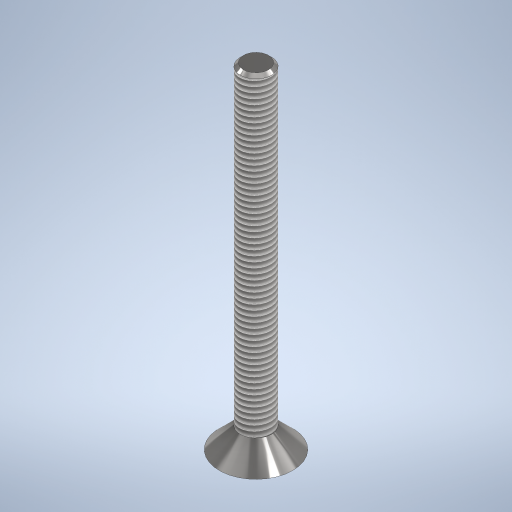
# Autodesk Inventor part: M3 30mm 십자나사
Saved by Autodesk Inventor 2023 (Build 270158000, 158)
## iProperties
Created: 2022-06-21
Part Number: M3 30mm 십자나사
Material: 일반
Document SubType Name: Modeling
Designer: user
Density: 1 g/cm^3
Appearance: 기본값
Author: user
Autodesk Inventor part; units mm, degrees
ref_plane "YZ Plane" through (0, 0, 0) normal (1, 0, 0) x (0, 1, 0)
ref_plane "XZ Plane" through (0, 0, 0) normal (0, 1, 0) x (-1, 0, 0)
ref_plane "XY Plane" through (0, 0, 0) normal (0, 0, 1) x (1, 0, 0)
sketch "스케치1" plane through (0, 0, 0) normal (0, 0, 1) x (1, 0, 0)
  line L0 (0, 0) -> (0, 30)
  line L1 (0, 30) -> (1.5, 30)
  line L2 (1.5, 30) -> (1.5, 0)
  line L3 (0, -2) -> (3.5, -2)
  line L4 (3.5, -2) -> (1.5, 0)
  line L5 (0, 0) -> (0, -2)
  dimension "d0" = 30
  dimension "d1" = 7
  dimension "d2" = 3
  dimension "d3" = 45
  constraints: 12 end point, 2 perpendicular, 2 vertical, 1 horizontal, 1 horizontal alignment
  measures "d0" distance of L0.start L0.end
  measures "d1" diameter of L3.end L0
  measures "d2" diameter of L2 L0
  measures "d3" angle of L5 L4
revolve "회전1" add sketch "스케치1" angle 360 about axis through (0, 0, 0) along (0, 1, 0)
chamfer "모따기1" distance 0.3 angle 45 1 edges at (-1.5, 30, 0)
thread "스레드1" size "M3x0.5" class "6g" standard "ANSI Metric M Profile" full length
sketch "스케치2" plane through (0, -2, 0) normal (0, -1, 0) x (1, 0, 0)
  line L0 (-0.5, 2.5) -> (0.5, 2.5)
  line L1 (0.5, 2.5) -> (0.5, -2.5)
  line L2 (0.5, -2.5) -> (-0.5, -2.5)
  line L3 (-0.5, -2.5) -> (-0.5, 2.5)
  circle A0 centre (0, 0) radius 1.2 construction
  line L4 (-0.5, 2.5) -> (0.5, -2.5) construction
  line L5 (0.5, 2.5) -> (-0.5, -2.5) construction
  line L6 (-2.5, -0.5) -> (2.5, -0.5)
  line L7 (2.5, -0.5) -> (2.5, 0.5)
  line L8 (2.5, 0.5) -> (-2.5, 0.5)
  line L9 (-2.5, 0.5) -> (-2.5, -0.5)
  line L10 (-2.5, -0.5) -> (2.5, 0.5) construction
  line L11 (2.5, -0.5) -> (-2.5, 0.5) construction
  point P0 (-0.5, 0.5)
  point P1 (-0.5, -0.5)
  point P2 (0.5, -0.5)
  point P3 (0.5, 0.5)
  dimension "d10" = 1
  dimension "d11" = 5
  dimension "d12" = 5
  dimension "d13" = 1
  constraints: 24 end point, 4 midpoint, 4 parallel, 2 horizontal, 2 perpendicular
  measures "d10" distance of L1.end L2.end
  measures "d11" distance of L0.end L1.end
  measures "d12" distance of L8.end L7.end
  measures "d13" distance of L7.end L6.end
extrude "돌출1" cut sketch "스케치2" against normal blind 0.5
